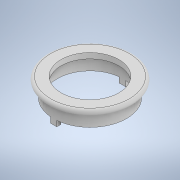
# Autodesk Inventor part: vez-rotate
Saved by Autodesk Inventor 2022 (Build 260153000, 153)
## iProperties
Created: 2022-11-30
Part Number: vez-rotate
Material: Generic
Document SubType Name: Modeling
Designer: matys
Density: 1 g/cm^3
Appearance: Default
Author: matys
Autodesk Inventor part; units mm, degrees
ref_plane "YZ Plane" through (0, 0, 0) normal (1, 0, 0) x (0, 1, 0)
ref_plane "XZ Plane" through (0, 0, 0) normal (0, 1, 0) x (-1, 0, 0)
ref_plane "XY Plane" through (0, 0, 0) normal (0, 0, 1) x (1, 0, 0)
sketch "Sketch1" plane through (0, 0, 0) normal (0, 1, 0) x (-1, 0, 0)
  circle A0 centre (0, 0) radius 30
  line L0 (30, 0) -> (33.5, 0)
  circle A1 centre (0, 0) radius 33.5
  dimension "d0" = 60
  dimension "d1" = 3.5
  constraints: 2 coincident, 2 end point, 2 horizontal alignment, 1 horizontal, 4 other
  measures "d1" distance of L0.start L0.end
extrude "Extrusion1" add sketch "Sketch1" along normal blind 12
sketch "Sketch2" plane through (0, 12, 0) normal (0, 1, 0) x (1, 0, 0)
  circle A0 centre (0, 0) radius 30 projected
  line L0 (0, -30) -> (0, -26.5)
  line L1 (0, -26.5) -> (0, -33.5)
  circle A1 centre (0, 0) radius 33.5 projected
  line L2 (0, -33.5) -> (0, -38.5)
  circle A2 centre (0, 0) radius 26.5
  circle A3 centre (0, 0) radius 38.5
  dimension "d4" = 3.5
  dimension "d5" = 5
  constraints: 6 end point, 4 vertical alignment, 2 coincident, 2 point on line, 1 vertical, 6 other
  measures "d4" distance of L0.start L0.end
  measures "d5" distance of L1.end L2.end
extrude "Extrusion2" add sketch "Sketch2" along normal blind 5 contours A0 | A1 | A3
sketch "Sketch3" plane through (0, 0, 0) normal (0, -1, 0) x (1, 0, 0)
  circle A0 centre (0, 0) radius 33.5 projected
  line L0 (0, 33.5) -> (0, -33.5)
  line L1 (3, 33.3654) -> (3, -33.5)
  line L2 (-3, 33.3654) -> (-3, -33.5)
  circle A1 centre (0, 0) radius 33.5
  circle A2 centre (0, 0) radius 30
  point P0 (3, 29.8496)
  point P1 (3, 33.3654)
  point P2 (-3, 33.3654)
  point P3 (-3, 29.8496)
  point P4 (3, -29.8496)
  point P5 (-3, -29.8496)
  point P6 (-3, -33.3654)
  point P7 (3, -33.3654)
  dimension "d8" = 3
  dimension "d9" = 3
  constraints: 6 end point, 4 point on circle, 2 centre point, 2 coincident, 2 parallel, 1 concentric, 1 vertical
  measures "d8" distance between parallel lines of L0 L1
  measures "d9" distance between parallel lines of L0 L2
extrude "Extrusion3" add sketch "Sketch3" along normal blind 5 contours L1 A2 L0 A0 | A0 L0 A2 L1 | L0 A2 L2 A0 | A0 L2 A2 L0
fillet "Fillet1" radius 2.5 2 edges at (-38.5, 12, 0) (-38.5, 17, 0)
body "Solid1"
